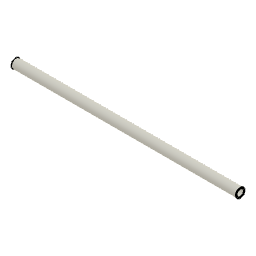
Version3EACCEnclsoure (Autodesk Fusion 360 archive; units mm, degrees)
design "PVC 3 ft pipe"
Autodesk Fusion 360 part; units mm, degrees
sketch "Sketch1" plane through (0, 0, 0) normal (1, 0, 0) x (0, 1, 0)
  circle A0 centre (0, 0) radius 12.7
  circle A1 centre (0, 0) radius 16.7005
  dimension "d1" = 25.4
  dimension "d2" = 33.401
  constraint coincident A0.centre A1.centre
  constraint concentric A0 A1
  measures "d1" diameter of A0
  measures "d2" diameter of A1
extrude "Extrude1" add sketch "Sketch1" along normal blind 825.5
equation "d3 = 30.5 in + 2 in"

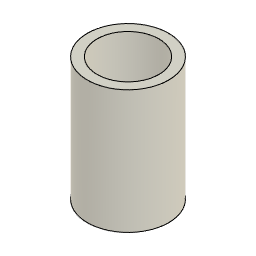
design "PVC 2 in pipe"
Autodesk Fusion 360 part; units mm, degrees
sketch "Sketch1" plane through (0, 0, 0) normal (0, 0, 1) x (1, 0, 0)
  circle A0 centre (0, 0) radius 12.7
  circle A1 centre (0, 0) radius 16.7005
  dimension "d1" = 25.4
  dimension "d2" = 33.401
  constraint coincident A0.centre A1.centre
  constraint concentric A0 A1
  measures "d1" diameter of A0
  measures "d2" diameter of A1
extrude "Extrude1" add sketch "Sketch1" along normal blind 50.8

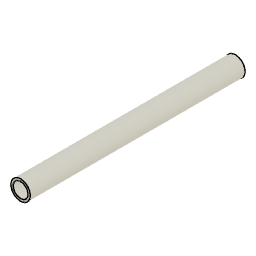
design "PVC 1.5 ft  pipe"
Autodesk Fusion 360 part; units mm, degrees
sketch "Sketch1" plane through (0, 0, 0) normal (0, 1, 0) x (1, 0, 0)
  circle A0 centre (0, 0) radius 12.7
  circle A1 centre (0, 0) radius 16.7005
  dimension "d1" = 25.4
  dimension "d2" = 33.401
  constraint coincident A0.centre A1.centre
  measures "d1" diameter of A0
  measures "d2" diameter of A1
extrude "Extrude1" add sketch "Sketch1" along normal blind 368.3

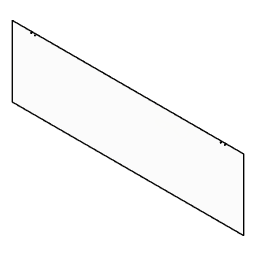
design "acrylic side"
Autodesk Fusion 360 part; units mm, degrees
sketch "Sketch1" plane through (0, 0, 0) normal (0, 1, 0) x (1, 0, 0)
  line L0 (0, 0) -> (914.4, 0)
  line L1 (914.4, 0) -> (914.4, -279.4)
  line L2 (914.4, -279.4) -> (0, -279.4)
  line L3 (0, -279.4) -> (0, 0)
  dimension "d1" = 914.4
  dimension "d2" = 279.4
  constraint horizontal L0
  constraint vertical L1
  constraint horizontal L2
  constraint vertical L3
  constraint coincident L0.start L3.end
  measures "d1" distance of L0.start L0.end
  measures "d2" distance of L0.start L2.end
extrude "Extrude1" add sketch "Sketch1" along normal blind 1.5875
sketch "Sketch2" plane through (0, 0, 0) normal (0, -1, 0) x (1, 0, 0)
  line L0 (914.4, 279.4) -> (0, 279.4)
  line L1 (0, 279.4) -> (0, 0)
  line L2 (0, 0) -> (914.4, 0)
  line L3 (914.4, 0) -> (914.4, 279.4)
  line L4 (0, 273.05) -> (914.4, 273.05) construction
  circle A0 centre (74.4888, 273.05) radius 1.8034
  circle A1 centre (90.3638, 273.05) radius 1.8034
  dimension "d5" = 6.35
  dimension "d6" = 3.6068
  dimension "d7" = 15.875
  dimension "d8" = 74.4888
  constraint coincident L1 L4.start
  constraint coincident L3 L4.end
  constraint perpendicular L3 L4
  constraint coincident L4 A0.centre
  constraint coincident L4 A1.centre
  constraint equal A0 A1
  measures "d5" distance of L0 L4
  measures "d6" diameter of A0
  measures "d7" distance of A0.centre A1.centre
  measures "d8" distance of L1 A0.centre
extrude "Extrude2" cut sketch "Sketch2" against normal blind 73.66 contours A0 | A1
ref_plane "WorkPlane1" through (457.2, 0.7937, 139.7) normal (1, 0, 0) x (0, 0, -1)
mirror "Mirror1" about plane through (457.2, 0.7937, 139.7) normal (1, 0, 0) of "Extrude2"
equation "d3 = ( 1 / 16 ) * 1 in"

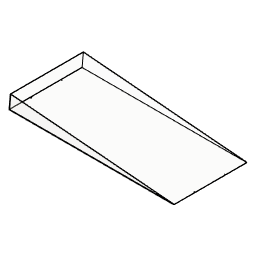
design "acrylic top pane"
Autodesk Fusion 360 part; units mm, degrees
sketch "Sketch1" plane through (0, 0, 0) normal (0, 0, 1) x (1, 0, 0)
  line L0 (0, 0) -> (818.261, 0) construction
  line L1 (818.261, 0) -> (818.261, 152.4) construction
  line L2 (818.261, 152.4) -> (0, 152.4) construction
  line L3 (0, 152.4) -> (0, 0) construction
  circle A0 centre (0, 0) radius 1.905
  circle A1 centre (818.261, 0) radius 1.5875
  line L4 (822.071, 156.21) -> (-3.81, 156.21) construction
  line L5 (-3.81, 156.21) -> (-3.81, -3.81)
  line L6 (-3.81, -3.81) -> (822.071, -3.81) construction
  line L7 (822.071, -3.81) -> (822.071, 156.21)
  line L8 (-3.81, -3.81) -> (822.071, -3.81) construction
  line L9 (822.071, -3.81) -> (822.071, -105.41)
  line L10 (822.071, -105.41) -> (-3.81, -105.41)
  line L11 (-3.81, -105.41) -> (-3.81, -3.81)
  line L12 (-3.81, 156.21) -> (822.071, 156.21) construction
  line L13 (822.071, 156.21) -> (822.071, 257.81)
  line L14 (822.071, 257.81) -> (-3.81, 257.81)
  line L15 (-3.81, 257.81) -> (-3.81, 156.21)
  circle A2 centre (0, 152.4) radius 1.5875
  circle A3 centre (818.261, 152.4) radius 1.5875
  dimension "d1" = 818.261
  dimension "d2" = 152.4
  dimension "d3" = 3.81
  dimension "d4" = 3.175
  dimension "d5" = 3.81
  dimension "d8" = 101.6
  dimension "d9" = 3.175
  dimension "d10" = 3.175
  constraint horizontal L0
  constraint vertical L1
  constraint horizontal L2
  constraint vertical L3
  constraint coincident L0.start L3.end
  constraint coincident L0.end L1.start
  constraint horizontal L8
  constraint vertical L9
  constraint horizontal L10
  constraint vertical L11
  constraint horizontal L12
  constraint vertical L13
  constraint horizontal L14
  constraint vertical L15
  constraint equal L9 L13
  constraint coincident L2.end L3.start
  constraint coincident L1.end L2.start
  measures "d1" distance of L0.start L0.end
  measures "d2" distance of L0.start L2.end
  measures "d3" diameter of A0
  measures "d4" diameter of A1
  measures "d8" distance of L6.end L9.end
  measures "d9" diameter of A2
  measures "d10" diameter of A3
extrude "Extrude1" add sketch "Sketch1" along normal blind 1.5875
sketch "Sketch2" plane through (0, -105.41, 0) normal (0, -1, 0) x (1, 0, 0)
  line L0 (-3.81, 0) -> (822.071, 0)
  line L1 (822.071, 0) -> (822.071, 1.5875)
  line L2 (822.071, 1.5875) -> (-3.81, 1.5875)
  line L3 (-3.81, 1.5875) -> (-3.81, 0)
  line L4 (2.0977, 71.1872) -> (822.071, 1.5875)
  line L5 (-3.81, 1.5875) -> (2.0977, 71.1872)
  dimension "d12" = 69.85
  constraint coincident L1.end L2.start
  constraint coincident L2.end L3.start
  constraint perpendicular L4 L5
  measures "d12" distance of L4.start L2.end
extrude "Extrude2" add sketch "Sketch2" along normal blind 1.5875
ref_plane "WorkPlane1" through (409.1305, 76.2, 0.7937) normal (0, 1, 0) x (-1, 0, 0)
mirror "Mirror1" about plane through (409.1305, 76.2, 0.7937) normal (0, 1, 0) of "Extrude2"
sketch "Sketch3" plane through (-3.9165, 0, 0.3324) normal (-0.996417, 0, 0.084576) x (0, -1, 0)
  line L0 (105.41, 71.1096) -> (105.41, 1.2596)
  line L1 (105.41, 1.2596) -> (106.9975, 1.2596)
  line L2 (106.9975, 1.2596) -> (106.9975, 71.1096)
  line L3 (106.9975, 71.1096) -> (105.41, 71.1096)
  line L4 (-257.81, 1.2596) -> (-257.81, 71.1096)
  line L5 (-257.81, 71.1096) -> (-259.3975, 71.1096)
  line L6 (-259.3975, 71.1096) -> (-259.3975, 1.2596)
  line L7 (-259.3975, 1.2596) -> (-257.81, 1.2596)
  line L8 (-257.81, 71.1096) -> (105.41, 71.1096)
  line L9 (105.41, 71.1096) -> (105.41, 1.2596)
  line L10 (105.41, 1.2596) -> (-257.81, 1.2596)
  line L11 (-257.81, 1.2596) -> (-257.81, 71.1096)
  constraint horizontal L8
  constraint vertical L9
  constraint horizontal L10
  constraint vertical L11
  constraint coincident L0.end L1.start
  constraint coincident L4.end L5.start
extrude "Extrude3" add sketch "Sketch3" against normal blind 1.5875 contours L0 L4 L8 L9 L10 L11
equation "d6 = ( 1 / 16 ) * 1 in"
equation "d13 = ( 1 / 16 ) * 1 in"
equation "d17 = -( 1 / 16 ) * 1 in"

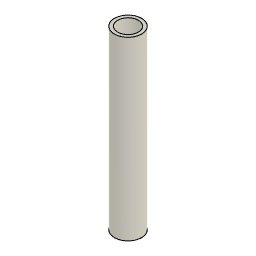
design "PVC 1 ft pipe"
Autodesk Fusion 360 part; units mm, degrees
sketch "Sketch1" plane through (0, 0, 0) normal (0, 0, 1) x (1, 0, 0)
  circle A0 centre (0, 0) radius 12.7
  circle A1 centre (0, 0) radius 16.7005
  dimension "d1" = 25.4
  dimension "d2" = 33.401
  constraint coincident A0.centre A1.centre
  measures "d1" diameter of A0
  measures "d2" diameter of A1
extrude "Extrude1" add sketch "Sketch1" along normal blind 215.9

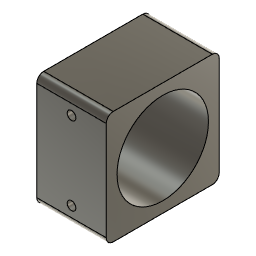
design "Pipe Mount"
Autodesk Fusion 360 part; units mm, degrees
sketch "Sketch2" plane through (0, 0, 0) normal (1, 0, 0) x (0, 1, 0)
  circle A0 centre (0, 0) radius 16.7005
  circle A1 centre (0, 0) radius 20.6375
  line L0 (-20.6375, 20.6375) -> (20.6375, 20.6375)
  line L1 (20.6375, 20.6375) -> (20.6375, -20.6375)
  line L2 (20.6375, -20.6375) -> (-20.6375, -20.6375)
  line L3 (-20.6375, -20.6375) -> (-20.6375, 20.6375)
  line L4 (-20.6375, 20.6375) -> (0, 0) construction
  line L5 (0, 0) -> (-20.6375, -20.6375) construction
  line L6 (20.6375, -20.6375) -> (0, 0) construction
  line L7 (20.6375, 20.6375) -> (0, 0) construction
  line L8 (-20.6375, -20.6375) -> (-14.5929, -14.5929)
  line L9 (20.6375, -20.6375) -> (14.5929, -14.5929)
  dimension "d1" = 33.401
  dimension "d2" = 41.275
  dimension "d3" = 41.275
  constraint coincident A0.centre A1.centre
  constraint concentric A0 A1
  constraint horizontal L0
  constraint vertical L1
  constraint horizontal L2
  constraint vertical L3
  constraint perpendicular L4 L5
  constraint perpendicular L5 L6
  constraint perpendicular L4 L7
  constraint coincident A1 L8.end
  constraint coincident L5 L8.end
  constraint coincident L6 L9.end
  constraint coincident A1 L9.end
  measures "d1" diameter of A0
  measures "d2" diameter of A1
  measures "d3" distance of L0.start L0.end
extrude "Extrude1" add sketch "Sketch2" along normal blind 25.4
sketch "Sketch3" plane through (0, 0, -20.6375) normal (0, 0, -1) x (1, 0, 0)
  line L0 (0, 20.6375) -> (0, -20.6375)
  line L1 (0, -20.6375) -> (25.4, -20.6375)
  line L2 (25.4, -20.6375) -> (25.4, 20.6375)
  line L3 (25.4, 20.6375) -> (0, 20.6375)
  line L4 (0, 14.2875) -> (25.4, 14.2875) construction
  line L5 (0, -14.2875) -> (25.4, -14.2875) construction
  circle A0 centre (3.81, 14.2875) radius 1.5875
  circle A1 centre (21.59, 14.2875) radius 1.5875
  circle A2 centre (3.81, -14.2875) radius 1.5875
  circle A3 centre (21.59, -14.2875) radius 1.5875
  dimension "d6" = 6.35
  dimension "d7" = 6.35
  dimension "d8" = 3.175
  dimension "d9" = 3.81
  dimension "d10" = 3.81
  dimension "d11" = 3.81
  dimension "d12" = 3.81
  constraint coincident L0 L4.start
  constraint coincident L2 L4.end
  constraint perpendicular L2 L4
  constraint coincident L0 L5.start
  constraint coincident L2 L5.end
  constraint perpendicular L2 L5
  constraint coincident L4 A0.centre
  constraint coincident L4 A1.centre
  constraint coincident L5 A2.centre
  constraint coincident L5 A3.centre
  constraint equal A2 A3
  constraint equal A1 A3
  constraint equal A0 A1
  measures "d6" distance of L3 L4
  measures "d7" distance of L1 L5
  measures "d8" diameter of A0
  measures "d9" distance of L4.start A0.centre
  measures "d10" distance of L4.end A1.centre
  measures "d11" horizontal distance of L0.end A2.centre
  measures "d12" distance of L5.end A3.centre
extrude "Extrude2" cut sketch "Sketch3" against normal blind 7.62 contours A0 | A1 | A2 | A3
sketch "Sketch4" plane through (0, -20.6375, 0) normal (0, -1, 0) x (1, 0, 0)
  line L0 (0, 20.6375) -> (0, -20.6375)
  line L1 (0, -20.6375) -> (25.4, -20.6375)
  line L2 (25.4, -20.6375) -> (25.4, 20.6375)
  line L3 (25.4, 20.6375) -> (0, 20.6375)
  line L4 (0, 16.8275) -> (25.4, 16.8275) construction
  line L5 (25.4, 16.8275) -> (25.4, -16.8275) construction
  line L6 (25.4, -16.8275) -> (0, -16.8275) construction
  line L7 (0, -16.8275) -> (0, 16.8275) construction
  line L8 (0, -20.6375) -> (25.4, -20.6375)
  circle A0 centre (8.89, 16.8275) radius 1.5875
  circle A1 centre (16.51, 16.8275) radius 1.5875
  circle A2 centre (8.89, -16.8275) radius 1.5875
  circle A3 centre (16.51, -16.8275) radius 1.5875
  dimension "d15" = 3.81
  dimension "d16" = 3.81
  dimension "d17" = 3.175
  dimension "d18" = 8.89
  dimension "d19" = 8.89
  dimension "d20" = 8.89
  dimension "d21" = 8.89
  constraint horizontal L4
  constraint vertical L5
  constraint horizontal L6
  constraint vertical L7
  constraint coincident L2 L5.end
  constraint coincident L0 L4.start
  constraint coincident L4 A0.centre
  constraint coincident L4 A1.centre
  constraint coincident L6 A2.centre
  constraint coincident L6 A3.centre
  constraint equal A0 A1
  constraint equal A1 A2
  constraint equal A2 A3
  measures "d15" distance of L6 L8
  measures "d16" distance of L3 L4
  measures "d17" diameter of A0
  measures "d18" distance of L4.start A0.centre
  measures "d19" distance of L4.end A1.centre
  measures "d20" distance of L6.end A2.centre
  measures "d21" distance of L5.end A3.centre
sketch "Sketch5" plane through (0, 20.6375, 0) normal (0, 1, 0) x (-1, 0, 0)
  line L0 (0, -20.6375) -> (0, 20.6375)
  line L1 (0, 20.6375) -> (-25.4, 20.6375)
  line L2 (-25.4, 20.6375) -> (-25.4, -20.6375)
  line L3 (-25.4, -20.6375) -> (0, -20.6375)
  line L4 (-12.7, 20.6375) -> (-12.7, -20.6375) construction
  circle A0 centre (-12.7, 14.2875) radius 1.5875
  circle A1 centre (-12.7, -14.2875) radius 1.5875
  dimension "d24" = 3.175
  dimension "d25" = 6.35
  dimension "d26" = 6.35
  constraint midpoint L1 L4.start
  constraint midpoint L3 L4.end
  constraint coincident L4 A0.centre
  constraint coincident L4 A1.centre
  constraint equal A0 A1
  measures "d24" diameter of A0
  measures "d25" distance of L4.end A1.centre
  measures "d26" distance of L1 A0.centre
extrude "Extrude4" cut sketch "Sketch5" against normal blind 7.62 contours A0 | A1
fillet "Fillet1" radius 2.54 4 edges at (12.7, -20.6375, 20.6375) (12.7, -20.6375, -20.6375) (12.7, 20.6375, -20.6375) (12.7, 20.6375, 20.6375)
ref_plane "WorkPlane1" through (12.7, 0, 0) normal (0, -1, 0) x (0, 0, -1)
mirror "Mirror1" about plane through (12.7, 0, 0) normal (0, -1, 0) of "Extrude4"
equation "d6 = d7"
equation "d8 = ( 1 / 8 ) * 1 in"
equation "d10 = d9"
equation "d11 = d9"
equation "d12 = d9"
equation "d16 = d15"
equation "d19 = d18"
equation "d20 = d18"
equation "d21 = d20"
equation "d26 = d25"

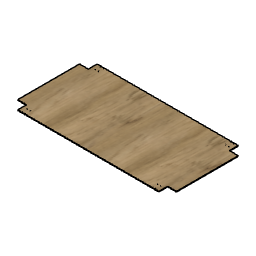
design "plywood 2"
Autodesk Fusion 360 part; units mm, degrees
sketch "Sketch1" plane through (0, 0, 0) normal (0, 0, 1) x (1, 0, 0)
  line L0 (0, 0) -> (914.4, 0)
  line L1 (914.4, 0) -> (914.4, 457.2)
  line L2 (914.4, 457.2) -> (0, 457.2)
  line L3 (0, 457.2) -> (0, 0)
  dimension "d1" = 457.2
  dimension "d2" = 914.4
  constraint horizontal L0
  constraint vertical L1
  constraint horizontal L2
  constraint vertical L3
  constraint coincident L0.start L3.end
  measures "d1" distance of L0.start L2.end
  measures "d2" distance of L0.start L0.end
extrude "Extrude1" add sketch "Sketch1" along normal blind 3.175
sketch "Sketch2" plane through (0, 0, 3.175) normal (0, 0, 1) x (-1, 0, 0)
  line L0 (0, -457.2) -> (0, 0) construction
  line L1 (0, 0) -> (-914.4, 0) construction
  line L2 (-914.4, 0) -> (-914.4, -457.2) construction
  line L3 (-914.4, -457.2) -> (0, -457.2) construction
  line L4 (-73.66, -453.39) -> (-91.44, -453.39) construction
  line L5 (-91.44, -453.39) -> (-91.44, -424.815) construction
  line L6 (-91.44, -424.815) -> (-73.66, -424.815) construction
  line L7 (-73.66, -424.815) -> (-73.66, -453.39) construction
  line L8 (-73.66, -32.385) -> (-91.44, -32.385) construction
  line L9 (-91.44, -32.385) -> (-91.44, -3.81) construction
  line L10 (-91.44, -3.81) -> (-73.66, -3.81) construction
  line L11 (-73.66, -3.81) -> (-73.66, -32.385) construction
  line L12 (-840.74, -453.39) -> (-840.74, -424.815) construction
  line L13 (-822.96, -32.385) -> (-840.74, -32.385) construction
  line L14 (-840.74, -32.385) -> (-840.74, -3.81) construction
  line L15 (-840.74, -3.81) -> (-822.96, -3.81) construction
  line L16 (-822.96, -3.81) -> (-822.96, -32.385) construction
  line L17 (-91.44, -453.39) -> (-840.74, -453.39) construction
  line L18 (-73.66, -424.815) -> (-73.66, -32.385) construction
  line L19 (-91.44, -3.81) -> (-822.96, -3.81) construction
  line L20 (-840.74, -32.385) -> (-840.74, -424.815) construction
  line L21 (-840.74, -424.815) -> (-822.96, -424.815) construction
  line L22 (-822.96, -424.815) -> (-822.96, -453.39) construction
  line L23 (-822.96, -453.39) -> (-840.74, -453.39) construction
  line L24 (-840.74, -453.39) -> (-840.74, -424.815) construction
  line L25 (0, -457.2) -> (-73.66, -453.39) construction
  line L26 (0, 0) -> (-73.66, -3.81) construction
  line L27 (-914.4, 0) -> (-840.74, -3.81) construction
  line L28 (-840.74, -453.39) -> (-914.4, -457.2) construction
  circle A0 centre (-73.66, -453.39) radius 1.5875
  circle A1 centre (-91.44, -453.39) radius 1.5875
  circle A2 centre (-91.44, -424.815) radius 1.5875
  circle A3 centre (-73.66, -424.815) radius 1.5875
  circle A4 centre (-73.66, -3.81) radius 1.5875
  circle A5 centre (-73.66, -32.385) radius 1.5875
  circle A6 centre (-91.44, -32.385) radius 1.5875
  circle A7 centre (-91.44, -3.81) radius 1.5875
  circle A8 centre (-822.96, -3.81) radius 1.5875
  circle A9 centre (-822.96, -32.385) radius 1.5875
  circle A10 centre (-840.74, -32.385) radius 1.5875
  circle A11 centre (-840.74, -3.81) radius 1.5875
  circle A12 centre (-822.96, -424.815) radius 1.5875
  circle A13 centre (-822.96, -453.39) radius 1.5875
  circle A14 centre (-840.74, -453.39) radius 1.5875
  circle A15 centre (-840.74, -424.815) radius 1.5875
  dimension "d6" = 767.08
  dimension "d7" = 449.58
  dimension "d8" = 17.78
  dimension "d9" = 28.575
  dimension "d10" = 3.175
  constraint horizontal L4
  constraint vertical L5
  constraint horizontal L6
  constraint vertical L7
  constraint horizontal L8
  constraint vertical L9
  constraint horizontal L10
  constraint vertical L11
  constraint vertical L12
  constraint horizontal L13
  constraint vertical L14
  constraint horizontal L15
  constraint vertical L16
  constraint perpendicular L8 L18
  constraint horizontal L21
  constraint vertical L22
  constraint horizontal L23
  constraint vertical L24
  constraint coincident L17 L22.end
  constraint coincident L0.start L3.end
  constraint coincident L0.end L1.start
  constraint coincident L1.end L2.start
  constraint coincident L2.end L3.start
  constraint equal L27 L28
  constraint equal L25 L26
  constraint perpendicular L17 L24
  constraint equal L25 L28
  constraint equal L13 L21
  constraint equal L8 L13
  constraint equal L6 L8
  constraint equal L5 L9
  constraint equal L5 L16
  constraint equal L16 L22
  constraint coincident L4.start L7.end
  constraint coincident L4.end L5.start
  constraint coincident L5.end L6.start
  constraint coincident L6.end L7.start
  constraint coincident L10.end L11.start
  constraint coincident L8.start L11.end
  constraint coincident L8.end L9.start
  constraint coincident L9.end L10.start
  constraint coincident L15.end L16.start
  constraint coincident L13.start L16.end
  constraint coincident L13.end L14.start
  constraint coincident L14.end L15.start
  constraint coincident L21.end L22.start
  constraint coincident L22.end L23.start
  constraint coincident L12.start L17.end
  constraint coincident L12.end L20.end
  constraint equal A13 A14
  constraint equal A14 A15
  constraint equal A12 A15
  constraint equal A9 A12
  constraint equal A9 A10
  constraint equal A10 A11
  constraint equal A8 A11
  constraint equal A7 A8
  constraint equal A5 A7
  constraint equal A4 A5
  constraint equal A4 A6
  constraint equal A1 A6
  constraint equal A1 A3
  constraint equal A2 A3
  constraint equal A0 A2
  measures "d6" distance of L18 L20
  measures "d7" distance of L17 L19
  measures "d8" distance of L12.end L21.end
  measures "d9" distance of L21.end L22.end
  measures "d10" diameter of A0
extrude "Extrude2" cut sketch "Sketch2" against normal blind 12.7
sketch "Sketch3" plane through (0, 0, 3.175) normal (0, 0, 1) x (-1, 0, 0)
  circle A0 centre (-91.44, -424.815) radius 1.5875
  circle A1 centre (-822.96, -453.39) radius 1.5875
  circle A2 centre (-822.96, -32.385) radius 1.5875
  circle A3 centre (-91.44, -3.81) radius 1.5875
  circle A4 centre (-73.66, -32.385) radius 1.5875
  circle A5 centre (-822.96, -3.81) radius 1.5875
  circle A6 centre (-822.96, -424.815) radius 1.5875
  circle A7 centre (-73.66, -453.39) radius 1.5875
  circle A8 centre (-73.66, -424.815) radius 1.5875
  circle A9 centre (-840.74, -453.39) radius 1.5875
  circle A10 centre (-840.74, -32.385) radius 1.5875
  circle A11 centre (-73.66, -3.81) radius 1.5875
  circle A12 centre (-91.44, -32.385) radius 1.5875
  circle A13 centre (-840.74, -3.81) radius 1.5875
  circle A14 centre (-840.74, -424.815) radius 1.5875
  circle A15 centre (-91.44, -453.39) radius 1.5875
  line L0 (0, -457.2) -> (0, 0)
  line L1 (0, 0) -> (-914.4, 0)
  line L2 (-914.4, 0) -> (-914.4, -457.2)
  line L3 (-914.4, -457.2) -> (0, -457.2)
  line L4 (0, -457.2) -> (-50.8, -457.2)
  line L5 (-50.8, -457.2) -> (-50.8, -406.4)
  line L6 (-50.8, -406.4) -> (0, -406.4)
  line L7 (0, -406.4) -> (0, -457.2)
  line L8 (0, 0) -> (-50.8, 0)
  line L9 (-50.8, 0) -> (-50.8, -50.8)
  line L10 (-50.8, -50.8) -> (0, -50.8)
  line L11 (0, -50.8) -> (0, 0)
  line L12 (-914.4, 0) -> (-863.6, 0)
  line L13 (-863.6, 0) -> (-863.6, -50.8)
  line L14 (-863.6, -50.8) -> (-914.4, -50.8)
  line L15 (-914.4, -50.8) -> (-914.4, 0)
  line L16 (-914.4, -457.2) -> (-863.6, -457.2)
  line L17 (-863.6, -457.2) -> (-863.6, -406.4)
  line L18 (-863.6, -406.4) -> (-914.4, -406.4)
  line L19 (-914.4, -406.4) -> (-914.4, -457.2)
  dimension "d13" = 50.8
  constraint horizontal L4
  constraint vertical L5
  constraint horizontal L6
  constraint vertical L7
  constraint coincident L0.start L3.end
  constraint horizontal L8
  constraint vertical L9
  constraint horizontal L10
  constraint vertical L11
  constraint coincident L0.end L1.start
  constraint horizontal L12
  constraint vertical L13
  constraint horizontal L14
  constraint vertical L15
  constraint coincident L1.end L2.start
  constraint horizontal L16
  constraint vertical L17
  constraint horizontal L18
  constraint vertical L19
  constraint coincident L2.end L3.start
  constraint equal L17 L18
  constraint equal L14 L18
  constraint equal L13 L14
  constraint equal L9 L13
  constraint equal L9 L10
  constraint equal L6 L10
  constraint equal L5 L6
  measures "d13" distance of L4.end L5.end
extrude "Extrude3" cut sketch "Sketch3" against normal blind 25.4 contours L0 L3 L4 L5 L6 L7 | L0 L1 L8 L9 L10 L11 | L2 L3 L16 L17 L18 L19 | L1 L2 L12 L13 L14 L15
equation "d3 = ( 1 / 8 ) * 1 in"

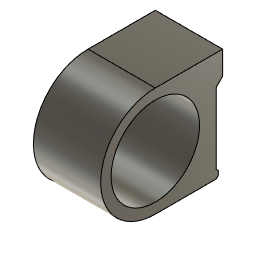
design "hinge mount"
Autodesk Fusion 360 part; units mm, degrees
sketch "Sketch1" plane through (0, 0, 0) normal (1, 0, 0) x (0, 1, 0)
  circle A0 centre (0, 0) radius 16.7005
  circle A1 centre (0, 0) radius 20.6375
  line L0 (0, 20.6375) -> (25.4, 20.6375)
  line L1 (25.4, 20.6375) -> (25.4, -20.6375)
  line L2 (25.4, -20.6375) -> (0, -20.6375)
  line L3 (0, -20.6375) -> (0, 20.6375) construction
  dimension "d1" = 33.401
  dimension "d2" = 41.275
  dimension "d10" = 25.4
  constraint coincident A0.centre A1.centre
  constraint concentric A0 A1
  constraint horizontal L0
  constraint vertical L1
  constraint horizontal L2
  constraint vertical L3
  constraint coincident A1 L0.start
  constraint tangent A1 L0
  constraint coincident A1 L2.end
  measures "d1" diameter of A0
  measures "d2" diameter of A1
  measures "d10" distance of A0.centre L1
extrude "Extrude1" add sketch "Sketch1" along normal blind 25.4
sketch "Sketch2" plane through (0, 25.4, 0) normal (0, 1, 0) x (-1, 0, 0)
  line L0 (0, -20.6375) -> (0, 20.6375)
  line L1 (0, 20.6375) -> (-25.4, 20.6375)
  line L2 (-25.4, 20.6375) -> (-25.4, -20.6375)
  line L3 (-25.4, -20.6375) -> (0, -20.6375)
  circle A0 centre (-20.1068, 17.2847) radius 1.8034
  circle A1 centre (-4.2318, 17.2847) radius 1.8034
  line L4 (-20.1068, 17.2847) -> (-4.2318, 17.2847) construction
  line L5 (-25.4, -20.6375) -> (-20.1068, 17.2847) construction
  line L6 (-4.2318, 17.2847) -> (0, -20.7706) construction
  dimension "d5" = 3.6068
  dimension "d6" = 15.875
  dimension "d11" = 3.3528
  constraint equal A0 A1
  constraint coincident A0.centre L4.start
  constraint coincident A1.centre L4.end
  constraint parallel L3 L4
  constraint coincident L2.end L3.start
  constraint coincident L0 L6.end
  constraint equal L5 L6
  measures "d5" diameter of A0
  measures "d6" distance of A0.centre A1.centre
  measures "d11" distance of L1 L4
extrude "Extrude2" cut sketch "Sketch2" against normal blind 7.62 contours A0 | A1
sketch "Sketch3" plane through (25.4, 0, 0) normal (1, 0, 0) x (0, 1, 0)
  circle A0 centre (0, 0) radius 16.7005
  line L0 (0, -20.6375) -> (25.4, -20.6375)
  line L1 (25.4, -20.6375) -> (25.4, 20.6375)
  line L2 (25.4, 20.6375) -> (0, 20.6375)
  arc A1 (0, 20.6375) -> (0, -20.6375) centre (0, 0) ccw
  line L3 (25.4, -20.6375) -> (23.0187, -20.6375)
  line L4 (23.0187, -20.6375) -> (23.0187, 11.7475)
  line L5 (23.0187, 11.7475) -> (25.4, 11.7475)
  line L6 (25.4, 11.7475) -> (25.4, -20.6375)
  line L7 (23.0187, -20.6375) -> (25.4, -20.6375)
  line L8 (25.4, -20.6375) -> (25.4, -18.2562)
  line L9 (25.4, -18.2562) -> (23.0187, -18.2562)
  line L10 (23.0187, -18.2562) -> (23.0187, -20.6375)
  line L11 (25.4, -18.2562) -> (23.8125, -18.2562)
  line L12 (23.8125, -18.2562) -> (23.8125, -20.6375)
  line L13 (23.8125, -20.6375) -> (25.4, -20.6375)
  line L14 (25.4, -20.6375) -> (25.4, -18.2562)
  dimension "d12" = 8.89
  dimension "d13" = 2.3813
  dimension "d18" = 0.7937
  constraint horizontal L3
  constraint vertical L4
  constraint horizontal L5
  constraint vertical L6
  constraint coincident L0.end L1.start
  constraint horizontal L7
  constraint vertical L8
  constraint horizontal L9
  constraint vertical L10
  constraint coincident L6 L8.end
  constraint equal L8 L9
  constraint horizontal L11
  constraint vertical L12
  constraint horizontal L13
  constraint vertical L14
  constraint coincident L7 L12.end
  measures "d12" distance of L2 L5
  measures "d13" distance of L0.end L3.end
  measures "d18" distance of L4 L12
extrude "Extrude3" cut sketch "Sketch3" against normal blind 62.23 contours L0 L1 L3 L6 L7 L8 L9 L11 L12 L13 L14 | L1 L4 L5 L6 L9 L11
chamfer "Chamfer1" distance 2.3813 angle 45 1 edges at (12.7, 23.0187, 11.7475)
chamfer "Chamfer1" distance 0.7937 angle 45 1 edges at (12.7, 23.0187, -18.2562)
chamfer "Chamfer1" distance 0.7937 angle 45 1 edges at (12.7, 23.8125, -20.6375)
equation "d13 = ( 3 / 32 ) * 1 in"
equation "d16 = ( 3 / 32 ) * 1 in"
equation "d17 = ( 1 / 32 ) * 1 in"
equation "d18 = ( 1 / 32 ) * 1 in"
equation "d19 = ( 1 / 32 ) * 1 in"
